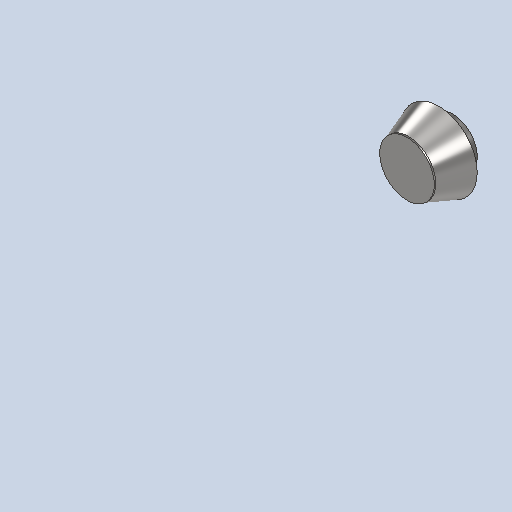
# Autodesk Inventor part: srb_thrusters_and_vectors
Saved by Autodesk Inventor 2024 (Build 280153000, 153)
## iProperties
Created: 2023-06-07
Part Number: srb_thrusters_and_vectors
Material: Steel, Mild
Document SubType Name: Modeling
Designer: tamiz
Density: 7.85 g/cm^3
Appearance: Semi-Polished
Author: tamiz
Autodesk Inventor part; units mm, degrees
ref_plane "YZ Plane" through (0, 0, 0) normal (1, 0, 0) x (0, 1, 0)
ref_plane "Work Plane3" through (0, 0, 17526) normal (0, 0, 1) x (1, 0, 0)
sketch "Sketch7" plane through (0, 0, 17526) normal (0, 0, 1) x (1, 0, 0)
  point P0 (0, 0)
ref_plane "Work Plane2" through (0, 0, -17526) normal (0, 0, -1) x (-1, 0, 0)
sketch "Sketch9" plane through (0, 0, -17526) normal (0, 0, -1) x (-1, 0, 0)
  circle A0 centre (0, 0) radius 2743.2
  constraints: 1 centre point, 1 coincident
extrude "Extrusion5" add sketch "Sketch9" along normal blind 152.4
sketch "Sketch11" plane through (0, 0, -17678.4) normal (0, 0, -1) x (-1, 0, 0)
  circle A0 centre (0, 0) radius 2743.2
  constraints: 1 centre point, 1 coincident
extrude "Extrusion7" add sketch "Sketch11" along normal blind 3048 draft 20
ref_plane "Work Plane4" through (0, 0, -17678.4) normal (0, 0, 1) x (1, 0, 0)
sketch "Sketch12" plane through (0, 0, -17678.4) normal (0, 0, 1) x (1, 0, 0)
  circle A0 centre (0, 0) radius 228.6
  dimension "d36" = 457.2
  constraints: 1 centre point, 1 coincident
  measures "d36" diameter of A0
extrude "Extrusion8" cut sketch "Sketch12" against normal blind 3048 draft 45
sketch "Sketch13" plane through (0, 0, 0) normal (1, 0, 0) x (0, 1, 0)
  line L0 (0, -17526) -> (0, -19964.4)
  arc A0 (1905.4646, -19981.2236) -> (2514.6, -19964.4) centre (2209.8, -19964.4) ccw
  line L1 (1905.4646, -19981.2236) -> (4118.293, -19981.2236) construction
  line L2 (2478.1868, -22118.6516) -> (1905.4646, -19981.2236)
  line L3 (2478.1868, -22118.6516) -> (2242.6554, -22181.762)
  line L4 (2242.6554, -22181.762) -> (1331.5059, -18781.3059)
  line L5 (2514.6, -19964.4) -> (1331.5059, -18781.3059)
  point P0 (0, 0)
  point P1 (1937.8261, -20101.998)
  dimension "d39" = 2438.4
  constraints: 12 end point, 2 point on circle, 1 centre point, 1 horizontal, 1 vertical
  measures "d39" distance of L0.start L0.end
revolve "Revolution5" add sketch "Sketch13" angle 360 about axis through (0, 0, -17526) along (0, 0, -1)
body "Solid1"
